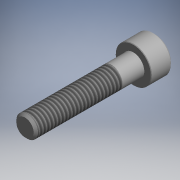
# Autodesk Inventor part: DIN-912 - M6x30(F)
Saved by Autodesk Inventor 2017.3 (Build 213256000, 256)
## iProperties
Part Number: DIN-912 - M6x30(F)
Material: Generic
Catalog Web Link: www.cadenas.de
Description: DIN-912-Cylinder screw
Vendor: FESTO
Document SubType Name: Modeling
Designer: partserver
Manufacturer: FESTO
Mass: 1.23562 g
Surface Area: 9.41163 cm^2
Volume: 1.23562 cm^3
Density: 1 g/cm^3
Appearance: PSOLRGB-192-192-192
Category: PARTsolutions
Company: FESTO
Title: DIN-912 - M6x30(F)
Author: Cadenas PARTsolutions
Comments: Cylinder screw
PSOL_IDENT_0: {$CADENAS_DATA\23d-libs\festo\zyl_zubeh\d912\din_912.prj},178 {VTYP=3D},{NB=DIN-912 - M6x30(F)},{LIN
PSOL_IDENT_1: A=DIN-912 - M6x30(F)},{NN=DIN-912},{DATE=01.07.2020 05:33:41},{GEOMDATE=01.07.2020 05:33:34},{VERSIO
PSOL_IDENT_2: N=},{LINEID=500},{WBVAR=},{WBNUMERIC=}  {NB=DIN-912 - M6x30(F)},{LINA=DIN-912 - M6x30(F)},{KT=X},{ID
PSOL_IDENT_3: NR=},{GEW=M6},{DG=6.000},{P=1.000},{L=30.000},{B=24.000},{FORM=0},{GKD=4.773},{DK=10.000},{DADIN=6.8
PSOL_IDENT_4: 00},{DS=6.000},{E=5.720},{LF=0.680},{K=6.000},{R=0.250},{S=5.000},{T=3.000},{V=0.600},{DW=9.380},{W=
PSOL_IDENT_5: 2.300},{NENN=M6x30},{DA=6.1},{BL=24}
NB: DIN-912 - M6x30(F)
NN: DIN-912
NT: Cylinder screw
NBSYN: DIN-912 - $NENN.(F)
LINA: DIN-912 - M6x30(F)
CATALOG: Festo
ROWDESC: M6x30
GEW: M6
DG: 6
P: 1
L: 30
B: 24
FORM: 0
GKD: 4.773
DK: 10
DADIN: 6.8
DS: 6
E: 5.72
LF: 0.68
K: 6
R: 0.25
S: 5
T: 3
V: 0.6
DW: 9.38
W: 2.3
SUPPLIER: FESTO
ARTICLENO: DIN-912 - M6x30(F)
BOMINFO: DIN-912 - M6x30(F)
CREATOR: CADENAS GmbH
Autodesk Inventor part; units mm, degrees
sketch "Sketch_1" plane through (0, 0, 0) normal (0, 0, 1) x (1, 0, 0)
  line L0 (0, -30) -> (0, 6)
  line L1 (0, 1.5566) -> (2.5, 3)
  line L2 (2.5, 3) -> (2.5, 5.6132)
  line L3 (2.5, 5.6132) -> (2.8868, 6)
  line L4 (2.8868, 6) -> (4.4, 6)
  line L5 (4.4, 6) -> (5, 5.4)
  line L6 (5, 5.4) -> (5, 0.15)
  line L7 (5, 0.15) -> (4.85, 0)
  line L8 (4.85, 0) -> (3.05, 0)
  line L9 (3.05, 0) -> (3, -0.68)
  line L10 (3, -0.68) -> (3, -29.3865)
  line L11 (3, -29.3865) -> (2.3865, -30)
  line L12 (2.3865, -30) -> (0, -30)
  line L13 (0, -30) -> (0, 1.5566)
  constraints: 28 end point
revolve "Revolution1" add sketch "Sketch_1" angle 360 about axis through (0, -30, 0) along (0, -1, 0)
thread "Thread1" size "M6x1" class "6g" standard "ISO Metric profile" length 23.3865
sketch "Sketch_2" plane through (0, 6, 0) normal (0, 1, 0) x (1, 0, 0)
  line L0 (-2.5, -1.4434) -> (0, -2.8868)
  line L1 (0, -2.8868) -> (2.5, -1.4434)
  line L2 (2.5, -1.4434) -> (2.5, 1.4434)
  line L3 (2.5, 1.4434) -> (0, 2.8868)
  line L4 (0, 2.8868) -> (-2.5, 1.4434)
  line L5 (-2.5, 1.4434) -> (-2.5, -1.4434)
  constraints: 12 end point
extrude "Extrusion1" cut sketch "Sketch_2" against normal blind 3
ref_plane "ANBAU_XY" through (0, 0, 0) normal (0, 1, 0) x (1, 0, 0)
ref_plane "ANBAU_YZ" through (0, 0, 0) normal (1, 0, 0) x (0, 0, -1)
ref_plane "ANBAU_ZX" through (0, 0, 0) normal (0, 0, -1) x (0, 1, 0)
ref_plane "Schraube_XY" through (0, 0, 0) normal (0, 1, 0) x (1, 0, 0)
ref_plane "Schraube_YZ" through (0, 0, 0) normal (1, 0, 0) x (0, 0, -1)
ref_plane "Schraube_ZX" through (0, 0, 0) normal (0, 0, -1) x (0, 1, 0)
ref_plane "insert_XY" through (0, 0, 0) normal (0, 1, 0) x (1, 0, 0)
ref_plane "insert_YZ" through (0, 0, 0) normal (1, 0, 0) x (0, 0, -1)
ref_plane "insert_ZX" through (0, 0, 0) normal (0, 0, -1) x (0, 1, 0)
ref_plane "schrauben_punkt_XY" through (0, -30, 0) normal (0, 1, 0) x (1, 0, 0)
ref_plane "schrauben_punkt_YZ" through (0, -30, 0) normal (1, 0, 0) x (0, 0, -1)
ref_plane "schrauben_punkt_ZX" through (0, -30, 0) normal (0, 0, -1) x (0, 1, 0)
body "Solid1"
